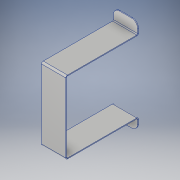
# Autodesk Inventor part: Handle
Saved by Autodesk Inventor 2019 (Build 230136000, 136)
## iProperties
Created: 2020-03-03
Part Number: Handle
Material: Aluminum 6061
Document SubType Name: Sheet Metal
Designer: student
Density: 2.7 g/cm^3
Flat Pattern Width: 2.54 cm
Flat Pattern Length: 24.7819 cm
Flat Pattern Area: 62.9461 cm^2
Sheet Metal Rule: Default
Sheet Metal Width: 1.000 in
Sheet Metal Length: 9.757 in
Sheet Metal Area: 9.757 in^2
Appearance: Aluminum - Flat
Author: student
Autodesk Inventor part; units mm, degrees
ref_plane "YZ Plane" through (0, 0, 0) normal (1, 0, 0) x (0, 1, 0)
ref_plane "XZ Plane" through (0, 0, 0) normal (0, 1, 0) x (-1, 0, 0)
ref_plane "XY Plane" through (0, 0, 0) normal (0, 0, 1) x (1, 0, 0)
sketch "Sketch1" plane through (0, 0, 0) normal (0, 0, 1) x (1, 0, 0)
  line L0 (12.7, -38.1) -> (-12.7, -38.1)
  line L1 (-12.7, -38.1) -> (-12.7, 38.1)
  line L2 (-12.7, 38.1) -> (12.7, 38.1)
  line L3 (12.7, 38.1) -> (12.7, -38.1)
  line L4 (12.7, -38.1) -> (-12.7, 38.1) construction
  line L5 (-12.7, -38.1) -> (12.7, 38.1) construction
  point P0 (0, 0)
  dimension "d0" = 25.4
  dimension "d1" = 76.2
  measures "d0" distance of L1.end L2.end
  measures "d1" distance between parallel lines of L0 L2
extrude "Plate1" add sketch "Sketch1" along normal blind 0.889
sketch "Sketch2" plane through (12.7, 37.211, 0.889) normal (0, 1, 0) x (-1, 0, 0)
  line L0 (25.4, 0) -> (0, 0)
  line L1 (0, 0) -> (0, -76.2)
  line L2 (0, -76.2) -> (25.4, -76.2)
  line L3 (25.4, -76.2) -> (25.4, 0)
  constraints: 6 end point, 1 horizontal, 1 perpendicular, 1 vertical
edge flange "Flange1" height 76.2 angle 90 thickness 0.889 bend radius 0.889 thickness toward (0, 1, 0) relief tear relief width 0.889 relief depth 0.4445 corner gap 0.889 corner form 0 edges at (0, 38.1, 0) (0, -38.1, 0) wall of the first edge with corners at (-12.7, 37.211, 0.889) (12.7, 37.211, 0.889) (12.7, 37.211, -75.311) (-12.7, 37.211, -75.311)
bend "Bend1"
corner "Corner1"
sketch "Sketch3" plane through (-12.7, 37.211, -74.422) normal (0, 0, -1) x (-1, 0, 0)
  line L0 (-25.4, 0) -> (0, 0)
  line L1 (0, 0) -> (0, 12.7)
  line L2 (0, 12.7) -> (-25.4, 12.7)
  line L3 (-25.4, 12.7) -> (-25.4, 0)
  constraints: 6 end point, 1 horizontal, 1 perpendicular, 1 vertical
edge flange "Flange2" height 12.7 angle 90 thickness 0.889 bend radius 0.889 thickness toward (0, 0, -1) relief tear relief width 0.889 relief depth 0.4445 corner gap 0.889 corner form 0 edges at (0, 38.1, -75.311) (0, -38.1, -75.311) wall of the first edge with corners at (12.7, 37.211, -74.422) (-12.7, 37.211, -74.422) (-12.7, 49.911, -74.422) (12.7, 49.911, -74.422)
bend "Bend2"
corner "Corner2"
fillet "Corner Round1" radius 6.35 4 edges at (12.7, 49.911, -74.8665) (-12.7, 49.911, -74.8665) (12.7, -49.911, -74.8665) (-12.7, -49.911, -74.8665)
equation "\"d2\" = Thickness"
equation "\"d3\" = BendReliefWidth"
equation "\"d4\" = BendReliefDepth"
equation "\"d5\" = MinimumRemnant"
equation "\"d6\" = TransitionRadius"
equation "\"d9\" = BendRadius"
equation "\"d10\" = CornerReliefSize"
equation "\"d11\" = GapSize"
equation "\"d12\" = JacobiRadiusSize"
equation "\"d13\" = BendReliefWidth"
equation "\"d14\" = BendReliefDepth"
equation "\"d15\" = MinimumRemnant"
equation "\"d16\" = TransitionRadius"
equation "\"d19\" = BendRadius"
equation "\"d20\" = CornerReliefSize"
equation "\"d21\" = GapSize"
equation "\"d22\" = JacobiRadiusSize"
equation "\"BendRadius\" = Thickness"
equation "\"BendReliefWidth\" = Thickness"
equation "\"BendReliefDepth\" = 0.5 * Thickness"
equation "\"CornerReliefSize\" = 4 * Thickness"
equation "\"MinimumRemnant\" = 2 * Thickness"
equation "\"TransitionRadius\" = BendRadius"
equation "\"JacobiRadiusSize\" = Thickness"
equation "\"GapSize\" = Thickness"
equation "\"Thickness\" = 0.889"
body "Solid1"
